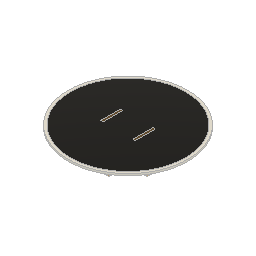
robotathon_field_2018 (Autodesk Fusion 360 design; units mm, degrees)
Autodesk Fusion 360 part; units mm, degrees
note: some values were not read from the file. Chosen so that the rebuilt part matches the saved one: which face or edge a step refers to.
sketch "Circle Sketch" plane through (0, 0, 0) normal (0, 1, 0) x (1, 0, 0)
  circle A0 centre (0, 0) radius 609.6
  dimension "d1" = 1219.2
  measures "d1" diameter of A0
extrude "Extrude1" add sketch "Circle Sketch" along normal mid plane 19.05 makes body 1
sketch "Split Face Sketch" plane through (0, 9.525, 0) normal (0, 1, 0) x (-1, 0, 0)
  circle A0 centre (0, 0) radius 609.6
  circle A1 centre (0, 0) radius 584.2
  line L0 (175.26, -101.6) -> (154.94, -101.6)
  line L1 (152.4, -99.06) -> (152.4, 99.06)
  line L2 (154.94, 101.6) -> (175.26, 101.6)
  line L3 (177.8, 99.06) -> (177.8, -99.06)
  line L4 (0, -609.6) -> (0, 609.6) construction
  line L5 (0, 0) -> (165.1, 0) construction
  arc A2 (175.26, -101.6) -> (177.8, -99.06) centre (175.26, -99.06) ccw
  arc A3 (152.4, -99.06) -> (154.94, -101.6) centre (154.94, -99.06) ccw
  arc A4 (154.94, 101.6) -> (152.4, 99.06) centre (154.94, 99.06) ccw
  arc A5 (177.8, 99.06) -> (175.26, 101.6) centre (175.26, 99.06) ccw
  arc A6 (-177.8, -99.06) -> (-175.26, -101.6) centre (-175.26, -99.06) ccw
  line L6 (-175.26, -101.6) -> (-154.94, -101.6)
  arc A7 (-154.94, -101.6) -> (-152.4, -99.06) centre (-154.94, -99.06) ccw
  arc A8 (-152.4, 99.06) -> (-154.94, 101.6) centre (-154.94, 99.06) ccw
  line L7 (-152.4, -99.06) -> (-152.4, 99.06)
  line L8 (-177.8, 99.06) -> (-177.8, -99.06)
  line L9 (-154.94, 101.6) -> (-175.26, 101.6)
  arc A9 (-175.26, 101.6) -> (-177.8, 99.06) centre (-175.26, 99.06) ccw
  dimension "d4" = 25.4
  dimension "d5" = 25.4
  dimension "d6" = 203.2
  dimension "d7" = 165.1
  dimension "d8" = 2.54
  measures "d4" distance of A0 A1
  measures "d7" distance of A0.centre
  measures "d8" radius of A2
split_face "SplitFace1" 1 faces at (74.2373, 9.525, 12.8232) by curves path "Split Face Sketch" along A1 on bodies 1
split_face "SplitFace2" 1 faces at (-60.9724, 9.525, -93.0704) by curves path "Split Face Sketch" along A2 L0 A3 L1 A4 L2 A5 L3 on bodies 1
split_face "SplitFace3" 1 faces at (93.1333, 9.525, 0) by curves path "Split Face Sketch" along L6 A7 L7 A8 L9 A9 L8 A6 on bodies 1
sketch "Standoff Sketch" plane through (0, -9.525, 0) normal (0, -1, 0) x (1, 0, 0)
  circle A0 centre (0, 0) radius 609.6
  line L0 (-304.8, 498.384) -> (304.8, 498.384)
  line L1 (304.8, 498.384) -> (304.8, 409.484)
  line L2 (304.8, 409.484) -> (-304.8, 409.484)
  line L3 (-304.8, 409.484) -> (-304.8, 498.384)
  line L4 (-304.8, 498.384) -> (304.8, 409.484) construction
  line L5 (0, 0) -> (0, 453.934) construction
  line L6 (304.8, 498.384) -> (318.0522, 520.0529) construction
  line L7 (-498.384, -304.8) -> (-498.384, 304.8)
  line L8 (-409.484, -304.8) -> (-498.384, -304.8)
  line L9 (-409.484, 304.8) -> (-409.484, -304.8)
  line L10 (-498.384, 304.8) -> (-409.484, 304.8)
  line L11 (304.8, -498.384) -> (-304.8, -498.384)
  line L12 (304.8, -409.484) -> (304.8, -498.384)
  line L13 (-304.8, -409.484) -> (304.8, -409.484)
  line L14 (-304.8, -498.384) -> (-304.8, -409.484)
  line L15 (498.384, 304.8) -> (498.384, -304.8)
  line L16 (409.484, 304.8) -> (498.384, 304.8)
  line L17 (409.484, -304.8) -> (409.484, 304.8)
  line L18 (498.384, -304.8) -> (409.484, -304.8)
  dimension "d9" = 88.9
  dimension "d10" = 609.6
  dimension "d11" = 25.4
  dimension "d13" = 360
extrude "Extrude1'" add sketch "Standoff Sketch" along normal blind 38.1 separate body contours L0 L1 L2 L3 | L7 L8 L9 L10 | L11 L12 L13 L14 | L15 L16 L17 L18 makes body 2 at (-101.6, -9.525, -439.1173) makes body 3 at (-439.1173, -9.525, -101.6) makes body 4 at (439.1173, -9.525, 101.6) makes body 5 at (101.6, -9.525, 439.1173) in component "Component"
component "Component" placed x (1, 0, 0) y (0, 1, 0) z (0, 0, 1) at (0, 0, 0)
named bodies: "Circle Extrude", "Standoff 1", "Standoff 2", "Standoff 3", "Standoff 4"
